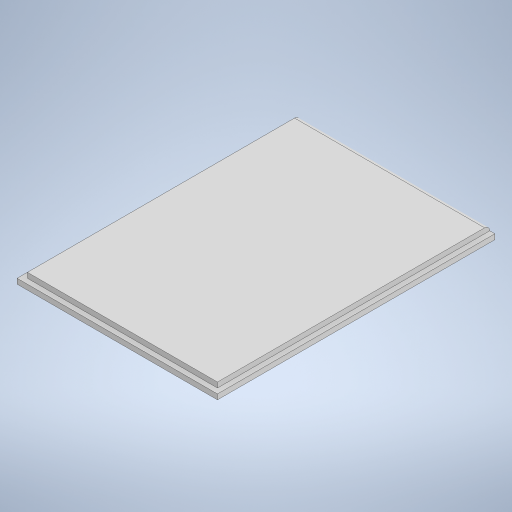
# Autodesk Inventor part: case_top
Saved by Autodesk Inventor 2024 (Build 280153000, 153)
## iProperties
Created: 2024-02-17
Part Number: case_top
Material: 一般
Document SubType Name: Modeling
Designer: Akio
Density: 1 g/cm^3
Appearance: 既定
Author: Akio
Autodesk Inventor part; units mm, degrees
ref_plane "YZ Plane" through (0, 0, 0) normal (1, 0, 0) x (0, 1, 0)
ref_plane "XZ Plane" through (0, 0, 0) normal (0, 1, 0) x (-1, 0, 0)
ref_plane "XY Plane" through (0, 0, 0) normal (0, 0, 1) x (1, 0, 0)
sketch "スケッチ1" plane through (0, 0, 0) normal (0, 1, 0) x (-1, 0, 0)
  line L0 (0, 0) -> (-39, 0)
  line L1 (-39, 0) -> (-39, -54)
  line L2 (-39, -54) -> (0, -54)
  line L3 (0, -54) -> (0, 0)
  dimension "d0" = 39
  dimension "d1" = 54
  constraints: 8 end point, 2 parallel, 1 horizontal, 1 perpendicular
  measures "d0" distance of L2.end L1.end
  measures "d1" distance of L1.end L0.end
extrude "押し出し1" add sketch "スケッチ1" along normal blind 1
sketch "スケッチ3" plane through (0, 1, 0) normal (0, 1, 0) x (1, 0, 0)
  line L0 (1, 1) -> (38, 1)
  line L1 (38, 1) -> (38, 54)
  line L2 (38, 54) -> (1, 54)
  line L3 (1, 54) -> (1, 1)
  line L4 (39, 54) -> (0, 54) projected
  line L5 (0, 54) -> (0, 0) projected
  dimension "d4" = 37
  dimension "d5" = 53
  dimension "d6" = 0
  dimension "d7" = 1
  constraints: 8 end point, 2 parallel, 1 horizontal, 1 perpendicular
  measures "d4" distance of L2.end L1.end
  measures "d5" distance of L1.end L0.end
  measures "d6" distance between parallel lines of L2 L4
  measures "d7" distance between parallel lines of L5 L3
extrude "押し出し2" add sketch "スケッチ3" along normal blind 1
fillet "フィレット1" radius 1 1 edges at (19.5, 2, -54)
